Autodesk Fusion 360 part; units mm, degrees
note: some values were not read from the file. Set by a fixed rule: which sketch regions a step uses.
(part 3 of 3)
  point P196 (12, -62.3538)
  point P197 (12, -62.3538)
  point P198 (24, -62.3538)
  point P199 (24, -62.3538)
  point P200 (26.5, -58.0237)
  point P201 (29, -62.3538)
  point P202 (24, -62.3538)
  point P203 (24, -62.3538)
  point P204 (36, -62.3538)
  point P205 (36, -62.3538)
  point P206 (38.5, -58.0237)
  point P207 (41, -62.3538)
  point P208 (36, -62.3538)
  point P209 (36, -62.3538)
  point P210 (48, -62.3538)
  point P211 (48, -62.3538)
  point P212 (50.5, -58.0237)
  point P213 (53, -62.3538)
  point P214 (48, -62.3538)
  point P215 (48, -62.3538)
  point P216 (60, -62.3538)
  point P217 (60, -62.3538)
  point P218 (62.5, -58.0237)
  point P219 (65, -62.3538)
  point P220 (60, -62.3538)
  point P221 (60, -62.3538)
  point P222 (72, -62.3538)
  point P223 (72, -62.3538)
  point P224 (74.5, -58.0237)
  point P225 (77, -62.3538)
  point P226 (72, -62.3538)
  point P227 (72, -62.3538)
  point P228 (-138, -51.9615)
  point P229 (-138, -51.9615)
  point P230 (-135.5, -47.6314)
  point P231 (-133, -51.9615)
  point P232 (-138, -51.9615)
  point P233 (-138, -51.9615)
  point P234 (-126, -51.9615)
  point P235 (-126, -51.9615)
  point P236 (-123.5, -47.6314)
  point P237 (-121, -51.9615)
  point P238 (-126, -51.9615)
  point P239 (-126, -51.9615)
  point P240 (-114, -51.9615)
  point P241 (-114, -51.9615)
  point P242 (-111.5, -47.6314)
  point P243 (-109, -51.9615)
  point P244 (-114, -51.9615)
  point P245 (-114, -51.9615)
  point P246 (-102, -51.9615)
  point P247 (-102, -51.9615)
  point P248 (-99.5, -47.6314)
  point P249 (-97, -51.9615)
  point P250 (-102, -51.9615)
  point P251 (-102, -51.9615)
  point P252 (-90, -51.9615)
  point P253 (-90, -51.9615)
  point P254 (-87.5, -47.6314)
  point P255 (-85, -51.9615)
  point P256 (-90, -51.9615)
  point P257 (-90, -51.9615)
  point P258 (-78, -51.9615)
  point P259 (-78, -51.9615)
  point P260 (-75.5, -47.6314)
  point P261 (-73, -51.9615)
  point P262 (-78, -51.9615)
  point P263 (-78, -51.9615)
  point P264 (-66, -51.9615)
  point P265 (-66, -51.9615)
  point P266 (-63.5, -47.6314)
  point P267 (-61, -51.9615)
  point P268 (-66, -51.9615)
  point P269 (-66, -51.9615)
  point P270 (-54, -51.9615)
  point P271 (-54, -51.9615)
  point P272 (-51.5, -47.6314)
  point P273 (-49, -51.9615)
  point P274 (-54, -51.9615)
  point P275 (-54, -51.9615)
  point P276 (-42, -51.9615)
  point P277 (-42, -51.9615)
  point P278 (-39.5, -47.6314)
  point P279 (-37, -51.9615)
  point P280 (-42, -51.9615)
  point P281 (-42, -51.9615)
  point P282 (-30, -51.9615)
  point P283 (-30, -51.9615)
  point P284 (-27.5, -47.6314)
  point P285 (-25, -51.9615)
  point P286 (-30, -51.9615)
  point P287 (-30, -51.9615)
  point P288 (-18, -51.9615)
  point P289 (-18, -51.9615)
  point P290 (-15.5, -47.6314)
  point P291 (-13, -51.9615)
  point P292 (-18, -51.9615)
  point P293 (-18, -51.9615)
  point P294 (-6, -51.9615)
  point P295 (-6, -51.9615)
  point P296 (-3.5, -47.6314)
  point P297 (-1, -51.9615)
  point P298 (-6, -51.9615)
  point P299 (-6, -51.9615)
  point P300 (6, -51.9615)
  point P301 (6, -51.9615)
  point P302 (8.5, -47.6314)
  point P303 (11, -51.9615)
  point P304 (6, -51.9615)
  point P305 (6, -51.9615)
  point P306 (18, -51.9615)
  point P307 (18, -51.9615)
  point P308 (20.5, -47.6314)
  point P309 (23, -51.9615)
  point P310 (18, -51.9615)
  point P311 (18, -51.9615)
  point P312 (30, -51.9615)
  point P313 (30, -51.9615)
  point P314 (32.5, -47.6314)
  point P315 (35, -51.9615)
  point P316 (30, -51.9615)
  point P317 (30, -51.9615)
  point P318 (42, -51.9615)
  point P319 (42, -51.9615)
  point P320 (44.5, -47.6314)
  point P321 (47, -51.9615)
  point P322 (42, -51.9615)
  point P323 (42, -51.9615)
  point P324 (54, -51.9615)
  point P325 (54, -51.9615)
  point P326 (56.5, -47.6314)
  point P327 (59, -51.9615)
  point P328 (54, -51.9615)
  point P329 (54, -51.9615)
  point P330 (66, -51.9615)
  point P331 (66, -51.9615)
  point P332 (68.5, -47.6314)
  point P333 (71, -51.9615)
  point P334 (66, -51.9615)
  point P335 (66, -51.9615)
  point P336 (78, -51.9615)
  point P337 (78, -51.9615)
  point P338 (80.5, -47.6314)
  point P339 (83, -51.9615)
  point P340 (78, -51.9615)
  point P341 (78, -51.9615)
  point P342 (-132, -41.5692)
  point P343 (-132, -41.5692)
  point P344 (-129.5, -37.2391)
  point P345 (-127, -41.5692)
  point P346 (-132, -41.5692)
  point P347 (-132, -41.5692)
  point P348 (-120, -41.5692)
  point P349 (-120, -41.5692)
  point P350 (-117.5, -37.2391)
  point P351 (-115, -41.5692)
  point P352 (-120, -41.5692)
  point P353 (-120, -41.5692)
  point P354 (-108, -41.5692)
  point P355 (-108, -41.5692)
  point P356 (-105.5, -37.2391)
  point P357 (-103, -41.5692)
  point P358 (-108, -41.5692)
  point P359 (-108, -41.5692)
  point P360 (-96, -41.5692)
  point P361 (-96, -41.5692)
  point P362 (-93.5, -37.2391)
  point P363 (-91, -41.5692)
  point P364 (-96, -41.5692)
  point P365 (-96, -41.5692)
  point P366 (-84, -41.5692)
  point P367 (-84, -41.5692)
  point P368 (-81.5, -37.2391)
  point P369 (-79, -41.5692)
  point P370 (-84, -41.5692)
  point P371 (-84, -41.5692)
  point P372 (-72, -41.5692)
  point P373 (-72, -41.5692)
  point P374 (-69.5, -37.2391)
  point P375 (-67, -41.5692)
  point P376 (-72, -41.5692)
  point P377 (-72, -41.5692)
  point P378 (-60, -41.5692)
  point P379 (-60, -41.5692)
  point P380 (-57.5, -37.2391)
  point P381 (-55, -41.5692)
  point P382 (-60, -41.5692)
  point P383 (-60, -41.5692)
  point P384 (-48, -41.5692)
  point P385 (-48, -41.5692)
  point P386 (-45.5, -37.2391)
  point P387 (-43, -41.5692)
  point P388 (-48, -41.5692)
  point P389 (-48, -41.5692)
  point P390 (-36, -41.5692)
  point P391 (-36, -41.5692)
  point P392 (-33.5, -37.2391)
  point P393 (-31, -41.5692)
  point P394 (-36, -41.5692)
  point P395 (-36, -41.5692)
  point P396 (-24, -41.5692)
  point P397 (-24, -41.5692)
  point P398 (-21.5, -37.2391)
  point P399 (-19, -41.5692)
  point P400 (-24, -41.5692)
  point P401 (-24, -41.5692)
  point P402 (-12, -41.5692)
  point P403 (-12, -41.5692)
  point P404 (-9.5, -37.2391)
  point P405 (-7, -41.5692)
  point P406 (-12, -41.5692)
  point P407 (-12, -41.5692)
  point P408 (0, -41.5692)
  point P409 (0, -41.5692)
  point P410 (2.5, -37.2391)
  point P411 (5, -41.5692)
  point P412 (0, -41.5692)
  point P413 (0, -41.5692)
  point P414 (12, -41.5692)
  point P415 (12, -41.5692)
  point P416 (14.5, -37.2391)
  point P417 (17, -41.5692)
  point P418 (12, -41.5692)
  point P419 (12, -41.5692)
  point P420 (24, -41.5692)
  point P421 (24, -41.5692)
  point P422 (26.5, -37.2391)
  point P423 (29, -41.5692)
  point P424 (24, -41.5692)
  point P425 (24, -41.5692)
  point P426 (36, -41.5692)
  point P427 (36, -41.5692)
  point P428 (38.5, -37.2391)
  point P429 (41, -41.5692)
  point P430 (36, -41.5692)
  point P431 (36, -41.5692)
  point P432 (48, -41.5692)
  point P433 (48, -41.5692)
  point P434 (50.5, -37.2391)
  point P435 (53, -41.5692)
  point P436 (48, -41.5692)
  point P437 (48, -41.5692)
  point P438 (60, -41.5692)
  point P439 (60, -41.5692)
  point P440 (62.5, -37.2391)
  point P441 (65, -41.5692)
  point P442 (60, -41.5692)
  point P443 (60, -41.5692)
  point P444 (72, -41.5692)
  point P445 (72, -41.5692)
  point P446 (74.5, -37.2391)
  point P447 (77, -41.5692)
  point P448 (72, -41.5692)
  point P449 (72, -41.5692)
  point P450 (84, -41.5692)
  point P451 (84, -41.5692)
  point P452 (86.5, -37.2391)
  point P453 (89, -41.5692)
  point P454 (84, -41.5692)
  point P455 (84, -41.5692)
  point P456 (-126, -31.1769)
  point P457 (-126, -31.1769)
  point P458 (-123.5, -26.8468)
  point P459 (-121, -31.1769)
  point P460 (-126, -31.1769)
  point P461 (-126, -31.1769)
  point P462 (-114, -31.1769)
  point P463 (-114, -31.1769)
  point P464 (-111.5, -26.8468)
  point P465 (-109, -31.1769)
  point P466 (-114, -31.1769)
  point P467 (-114, -31.1769)
  point P468 (-102, -31.1769)
  point P469 (-102, -31.1769)
  point P470 (-99.5, -26.8468)
  point P471 (-97, -31.1769)
  point P472 (-102, -31.1769)
  point P473 (-102, -31.1769)
  point P474 (-90, -31.1769)
  point P475 (-90, -31.1769)
  point P476 (-87.5, -26.8468)
  point P477 (-85, -31.1769)
  point P478 (-90, -31.1769)
  point P479 (-90, -31.1769)
  point P480 (-78, -31.1769)
  point P481 (-78, -31.1769)
  point P482 (-75.5, -26.8468)
  point P483 (-73, -31.1769)
  point P484 (-78, -31.1769)
  point P485 (-78, -31.1769)
  point P486 (-66, -31.1769)
  point P487 (-66, -31.1769)
  point P488 (-63.5, -26.8468)
  point P489 (-61, -31.1769)
  point P490 (-66, -31.1769)
  point P491 (-66, -31.1769)
  point P492 (-54, -31.1769)
  point P493 (-54, -31.1769)
  point P494 (-51.5, -26.8468)
  point P495 (-49, -31.1769)
  point P496 (-54, -31.1769)
  point P497 (-54, -31.1769)
  point P498 (-42, -31.1769)
  point P499 (-42, -31.1769)
  point P500 (-39.5, -26.8468)
  point P501 (-37, -31.1769)
  point P502 (-42, -31.1769)
  point P503 (-42, -31.1769)
  point P504 (-30, -31.1769)
  point P505 (-30, -31.1769)
  point P506 (-27.5, -26.8468)
  point P507 (-25, -31.1769)
  point P508 (-30, -31.1769)
  point P509 (-30, -31.1769)
  point P510 (-18, -31.1769)
  point P511 (-18, -31.1769)
  point P512 (-15.5, -26.8468)
  point P513 (-13, -31.1769)
  point P514 (-18, -31.1769)
  point P515 (-18, -31.1769)
  point P516 (-6, -31.1769)
  point P517 (-6, -31.1769)
  point P518 (-3.5, -26.8468)
  point P519 (-1, -31.1769)
  point P520 (-6, -31.1769)
  point P521 (-6, -31.1769)
  point P522 (6, -31.1769)
  point P523 (6, -31.1769)
  point P524 (8.5, -26.8468)
  point P525 (11, -31.1769)
  point P526 (6, -31.1769)
  point P527 (6, -31.1769)
  point P528 (18, -31.1769)
  point P529 (18, -31.1769)
  point P530 (20.5, -26.8468)
  point P531 (23, -31.1769)
  point P532 (18, -31.1769)
  point P533 (18, -31.1769)
  point P534 (30, -31.1769)
  point P535 (30, -31.1769)
  point P536 (32.5, -26.8468)
  point P537 (35, -31.1769)
  point P538 (30, -31.1769)
  point P539 (30, -31.1769)
  point P540 (42, -31.1769)
  point P541 (42, -31.1769)
  point P542 (44.5, -26.8468)
  point P543 (47, -31.1769)
  point P544 (42, -31.1769)
  point P545 (42, -31.1769)
  point P546 (54, -31.1769)
  point P547 (54, -31.1769)
  point P548 (56.5, -26.8468)
  point P549 (59, -31.1769)
  point P550 (54, -31.1769)
  point P551 (54, -31.1769)
  point P552 (66, -31.1769)
  point P553 (66, -31.1769)
  point P554 (68.5, -26.8468)
  point P555 (71, -31.1769)
  point P556 (66, -31.1769)
  point P557 (66, -31.1769)
  point P558 (78, -31.1769)
  point P559 (78, -31.1769)
  point P560 (80.5, -26.8468)
  point P561 (83, -31.1769)
  point P562 (78, -31.1769)
  point P563 (78, -31.1769)
  point P564 (90, -31.1769)
  point P565 (90, -31.1769)
  point P566 (92.5, -26.8468)
  point P567 (95, -31.1769)
  point P568 (90, -31.1769)
  point P569 (90, -31.1769)
  point P570 (-120, -20.7846)
  point P571 (-120, -20.7846)
  point P572 (-117.5, -16.4545)
  point P573 (-115, -20.7846)
  point P574 (-120, -20.7846)
  point P575 (-120, -20.7846)
  point P576 (-108, -20.7846)
  point P577 (-108, -20.7846)
  point P578 (-105.5, -16.4545)
  point P579 (-103, -20.7846)
  point P580 (-108, -20.7846)
  point P581 (-108, -20.7846)
  point P582 (-96, -20.7846)
  point P583 (-96, -20.7846)
  point P584 (-93.5, -16.4545)
  point P585 (-91, -20.7846)
  point P586 (-96, -20.7846)
  point P587 (-96, -20.7846)
  point P588 (-84, -20.7846)
  point P589 (-84, -20.7846)
  point P590 (-81.5, -16.4545)
  point P591 (-79, -20.7846)
  point P592 (-84, -20.7846)
  point P593 (-84, -20.7846)
  point P594 (-72, -20.7846)
  point P595 (-72, -20.7846)
  point P596 (-69.5, -16.4545)
  point P597 (-67, -20.7846)
  point P598 (-72, -20.7846)
  point P599 (-72, -20.7846)
  point P600 (-60, -20.7846)
  point P601 (-60, -20.7846)
  point P602 (-57.5, -16.4545)
  point P603 (-55, -20.7846)
  point P604 (-60, -20.7846)
  point P605 (-60, -20.7846)
  point P606 (-48, -20.7846)
  point P607 (-48, -20.7846)
  point P608 (-45.5, -16.4545)
  point P609 (-43, -20.7846)
  point P610 (-48, -20.7846)
  point P611 (-48, -20.7846)
  point P612 (-36, -20.7846)
  point P613 (-36, -20.7846)
  point P614 (-33.5, -16.4545)
  point P615 (-31, -20.7846)
  point P616 (-36, -20.7846)
  point P617 (-36, -20.7846)
  point P618 (-24, -20.7846)
  point P619 (-24, -20.7846)
  point P620 (-21.5, -16.4545)
  point P621 (-19, -20.7846)
  point P622 (-24, -20.7846)
  point P623 (-24, -20.7846)
  point P624 (-12, -20.7846)
  point P625 (-12, -20.7846)
  point P626 (-9.5, -16.4545)
  point P627 (-7, -20.7846)
  point P628 (-12, -20.7846)
  point P629 (-12, -20.7846)
  point P630 (0, -20.7846)
  point P631 (0, -20.7846)
  point P632 (2.5, -16.4545)
  point P633 (5, -20.7846)
  point P634 (0, -20.7846)
  point P635 (0, -20.7846)
  point P636 (12, -20.7846)
  point P637 (12, -20.7846)
  point P638 (14.5, -16.4545)
  point P639 (17, -20.7846)
  point P640 (12, -20.7846)
  point P641 (12, -20.7846)
  point P642 (24, -20.7846)
  point P643 (24, -20.7846)
  point P644 (26.5, -16.4545)
  point P645 (29, -20.7846)
  point P646 (24, -20.7846)
  point P647 (24, -20.7846)
  point P648 (36, -20.7846)
  point P649 (36, -20.7846)
  point P650 (38.5, -16.4545)
  point P651 (41, -20.7846)
  point P652 (36, -20.7846)
  point P653 (36, -20.7846)
  point P654 (48, -20.7846)
  point P655 (48, -20.7846)
  point P656 (50.5, -16.4545)
  point P657 (53, -20.7846)
  point P658 (48, -20.7846)
  point P659 (48, -20.7846)
  point P660 (60, -20.7846)
  point P661 (60, -20.7846)
  point P662 (62.5, -16.4545)
  point P663 (65, -20.7846)
  point P664 (60, -20.7846)
  point P665 (60, -20.7846)
  point P666 (72, -20.7846)
  point P667 (72, -20.7846)
  point P668 (74.5, -16.4545)
  point P669 (77, -20.7846)
  point P670 (72, -20.7846)
  point P671 (72, -20.7846)
  point P672 (84, -20.7846)
  point P673 (84, -20.7846)
  point P674 (86.5, -16.4545)
  point P675 (89, -20.7846)
  point P676 (84, -20.7846)
  point P677 (84, -20.7846)
  point P678 (96, -20.7846)
  point P679 (96, -20.7846)
  point P680 (98.5, -16.4545)
  point P681 (101, -20.7846)
  point P682 (96, -20.7846)
  point P683 (96, -20.7846)
  point P684 (-114, -10.3923)
  point P685 (-114, -10.3923)
  point P686 (-111.5, -6.0622)
  point P687 (-109, -10.3923)
  point P688 (-114, -10.3923)
  point P689 (-114, -10.3923)
  point P690 (-102, -10.3923)
  point P691 (-102, -10.3923)
  point P692 (-99.5, -6.0622)
  point P693 (-97, -10.3923)
  point P694 (-102, -10.3923)
  point P695 (-102, -10.3923)
  point P696 (-90, -10.3923)
  point P697 (-90, -10.3923)
  point P698 (-87.5, -6.0622)
  point P699 (-85, -10.3923)
  point P700 (-90, -10.3923)
  point P701 (-90, -10.3923)
  point P702 (-78, -10.3923)
  point P703 (-78, -10.3923)
  point P704 (-75.5, -6.0622)
  point P705 (-73, -10.3923)
  point P706 (-78, -10.3923)
  point P707 (-78, -10.3923)
  point P708 (-66, -10.3923)
  point P709 (-66, -10.3923)
  point P710 (-63.5, -6.0622)
  point P711 (-61, -10.3923)
  point P712 (-66, -10.3923)
  point P713 (-66, -10.3923)
  point P714 (-54, -10.3923)
  point P715 (-54, -10.3923)
  point P716 (-51.5, -6.0622)
  point P717 (-49, -10.3923)
  point P718 (-54, -10.3923)
  point P719 (-54, -10.3923)
  point P720 (-42, -10.3923)
  point P721 (-42, -10.3923)
  point P722 (-39.5, -6.0622)
  point P723 (-37, -10.3923)
  point P724 (-42, -10.3923)
  point P725 (-42, -10.3923)
  point P726 (-30, -10.3923)
  point P727 (-30, -10.3923)
  point P728 (-27.5, -6.0622)
  point P729 (-25, -10.3923)
  point P730 (-30, -10.3923)
  point P731 (-30, -10.3923)
  point P732 (-18, -10.3923)
  point P733 (-18, -10.3923)
  point P734 (-15.5, -6.0622)
  point P735 (-13, -10.3923)
  point P736 (-18, -10.3923)
  point P737 (-18, -10.3923)
  point P738 (-6, -10.3923)
  point P739 (-6, -10.3923)
  point P740 (-3.5, -6.0622)
  point P741 (-1, -10.3923)
  point P742 (-6, -10.3923)
  point P743 (-6, -10.3923)
  point P744 (6, -10.3923)
  point P745 (6, -10.3923)
  point P746 (8.5, -6.0622)
  point P747 (11, -10.3923)
  point P748 (6, -10.3923)
  point P749 (6, -10.3923)
  point P750 (18, -10.3923)
  point P751 (18, -10.3923)
  point P752 (20.5, -6.0622)
  point P753 (23, -10.3923)
  point P754 (18, -10.3923)
  point P755 (18, -10.3923)
  point P756 (30, -10.3923)
  point P757 (30, -10.3923)
  point P758 (32.5, -6.0622)
  point P759 (35, -10.3923)
  point P760 (30, -10.3923)
  point P761 (30, -10.3923)
  point P762 (42, -10.3923)
  point P763 (42, -10.3923)
  point P764 (44.5, -6.0622)
  point P765 (47, -10.3923)
  point P766 (42, -10.3923)
  point P767 (42, -10.3923)
  point P768 (54, -10.3923)
  point P769 (54, -10.3923)
  point P770 (56.5, -6.0622)
  point P771 (59, -10.3923)
  point P772 (54, -10.3923)
  point P773 (54, -10.3923)
  point P774 (66, -10.3923)
  point P775 (66, -10.3923)
  point P776 (68.5, -6.0622)
  point P777 (71, -10.3923)
  point P778 (66, -10.3923)
  point P779 (66, -10.3923)
  point P780 (78, -10.3923)
  point P781 (78, -10.3923)
  point P782 (80.5, -6.0622)
  point P783 (83, -10.3923)
  point P784 (78, -10.3923)
  point P785 (78, -10.3923)
  point P786 (90, -10.3923)
  point P787 (90, -10.3923)
  point P788 (92.5, -6.0622)
  point P789 (95, -10.3923)
  point P790 (90, -10.3923)
  point P791 (90, -10.3923)
  point P792 (102, -10.3923)
  point P793 (102, -10.3923)
  point P794 (104.5, -6.0622)
  point P795 (107, -10.3923)
  point P796 (102, -10.3923)
  point P797 (102, -10.3923)
  point P798 (-108, 0)
  point P799 (-108, 0)
  point P800 (-105.5, 4.3301)
  point P801 (-103, 0)
  point P802 (-108, 0)
  point P803 (-108, 0)
  point P804 (-96, 0)
  point P805 (-96, 0)
  point P806 (-93.5, 4.3301)
  point P807 (-91, 0)
  point P808 (-96, 0)
  point P809 (-96, 0)
  point P810 (-84, 0)
  point P811 (-84, 0)
  point P812 (-81.5, 4.3301)
  point P813 (-79, 0)
  point P814 (-84, 0)
  point P815 (-84, 0)
  point P816 (-72, 0)
  point P817 (-72, 0)
  point P818 (-69.5, 4.3301)
  point P819 (-67, 0)
  point P820 (-72, 0)
  point P821 (-72, 0)
  point P822 (-60, 0)
  point P823 (-60, 0)
  point P824 (-57.5, 4.3301)
  point P825 (-55, 0)
  point P826 (-60, 0)
  point P827 (-60, 0)
  point P828 (-48, 0)
  point P829 (-48, 0)
  point P830 (-45.5, 4.3301)
  point P831 (-43, 0)
  point P832 (-48, 0)
  point P833 (-48, 0)
  point P834 (-36, 0)
  point P835 (-36, 0)
  point P836 (-33.5, 4.3301)
  point P837 (-31, 0)
  point P838 (-36, 0)
  point P839 (-36, 0)
  point P840 (-24, 0)
  point P841 (-24, 0)
  point P842 (-21.5, 4.3301)
  point P843 (-19, 0)
  point P844 (-24, 0)
  point P845 (-24, 0)
  point P846 (-12, 0)
  point P847 (-12, 0)
  point P848 (-9.5, 4.3301)
  point P849 (-7, 0)
  point P850 (-12, 0)
  point P851 (-12, 0)
  point P852 (12, 0)
  point P853 (12, 0)
  point P854 (14.5, 4.3301)
  point P855 (17, 0)
  point P856 (12, 0)
  point P857 (12, 0)
  point P858 (24, 0)
  point P859 (24, 0)
  point P860 (26.5, 4.3301)
  point P861 (29, 0)
  point P862 (24, 0)
  point P863 (24, 0)
  point P864 (36, 0)
  point P865 (36, 0)
  point P866 (38.5, 4.3301)
  point P867 (41, 0)
  point P868 (36, 0)
  point P869 (36, 0)
  point P870 (48, 0)
  point P871 (48, 0)
  point P872 (50.5, 4.3301)
  point P873 (53, 0)
  point P874 (48, 0)
  point P875 (48, 0)
  point P876 (60, 0)
  point P877 (60, 0)
  point P878 (62.5, 4.3301)
  point P879 (65, 0)
  point P880 (60, 0)
  point P881 (60, 0)
  point P882 (72, 0)
  point P883 (72, 0)
  point P884 (74.5, 4.3301)
  point P885 (77, 0)
  point P886 (72, 0)
  point P887 (72, 0)
  point P888 (84, 0)
  point P889 (84, 0)
  point P890 (86.5, 4.3301)
  point P891 (89, 0)
  point P892 (84, 0)
  point P893 (84, 0)
  point P894 (96, 0)
  point P895 (96, 0)
  point P896 (98.5, 4.3301)
  point P897 (101, 0)
  point P898 (96, 0)
  point P899 (96, 0)
  point P900 (108, 0)
  point P901 (108, 0)
  point P902 (110.5, 4.3301)
  point P903 (113, 0)
  point P904 (108, 0)
  point P905 (108, 0)
  point P906 (-102, 10.3923)
  point P907 (-102, 10.3923)
  point P908 (-99.5, 14.7224)
  point P909 (-97, 10.3923)
  point P910 (-102, 10.3923)
  point P911 (-102, 10.3923)
  point P912 (-90, 10.3923)
  point P913 (-90, 10.3923)
  point P914 (-87.5, 14.7224)
  point P915 (-85, 10.3923)
  point P916 (-90, 10.3923)
  point P917 (-90, 10.3923)
  point P918 (-78, 10.3923)
  point P919 (-78, 10.3923)
  point P920 (-75.5, 14.7224)
  point P921 (-73, 10.3923)
  point P922 (-78, 10.3923)
  point P923 (-78, 10.3923)
  point P924 (-66, 10.3923)
  point P925 (-66, 10.3923)
  point P926 (-63.5, 14.7224)
  point P927 (-61, 10.3923)
  point P928 (-66, 10.3923)
  point P929 (-66, 10.3923)
  point P930 (-54, 10.3923)
  point P931 (-54, 10.3923)
  point P932 (-51.5, 14.7224)
  point P933 (-49, 10.3923)
  point P934 (-54, 10.3923)
  point P935 (-54, 10.3923)
  point P936 (-42, 10.3923)
  point P937 (-42, 10.3923)
  point P938 (-39.5, 14.7224)
  point P939 (-37, 10.3923)
  point P940 (-42, 10.3923)
  point P941 (-42, 10.3923)
  point P942 (-30, 10.3923)
  point P943 (-30, 10.3923)
  point P944 (-27.5, 14.7224)
  point P945 (-25, 10.3923)
  point P946 (-30, 10.3923)
  point P947 (-30, 10.3923)
  point P948 (-18, 10.3923)
  point P949 (-18, 10.3923)
  point P950 (-15.5, 14.7224)
  point P951 (-13, 10.3923)
  point P952 (-18, 10.3923)
  point P953 (-18, 10.3923)
  point P954 (-6, 10.3923)
  point P955 (-6, 10.3923)
  point P956 (-3.5, 14.7224)
  point P957 (-1, 10.3923)
  point P958 (-6, 10.3923)
  point P959 (-6, 10.3923)
  point P960 (6, 10.3923)
  point P961 (6, 10.3923)
  point P962 (8.5, 14.7224)
  point P963 (11, 10.3923)
  point P964 (6, 10.3923)
  point P965 (6, 10.3923)
  point P966 (18, 10.3923)
  point P967 (18, 10.3923)
  point P968 (20.5, 14.7224)
  point P969 (23, 10.3923)
  point P970 (18, 10.3923)
  point P971 (18, 10.3923)
  point P972 (30, 10.3923)
  point P973 (30, 10.3923)
  point P974 (32.5, 14.7224)
  point P975 (35, 10.3923)
  point P976 (30, 10.3923)
  point P977 (30, 10.3923)
  point P978 (42, 10.3923)
  point P979 (42, 10.3923)
  point P980 (44.5, 14.7224)
  point P981 (47, 10.3923)
  point P982 (42, 10.3923)
  point P983 (42, 10.3923)
  point P984 (54, 10.3923)
  point P985 (54, 10.3923)
  point P986 (56.5, 14.7224)
  point P987 (59, 10.3923)
  point P988 (54, 10.3923)
  point P989 (54, 10.3923)
  point P990 (66, 10.3923)
  point P991 (66, 10.3923)
  point P992 (68.5, 14.7224)
  point P993 (71, 10.3923)
  point P994 (66, 10.3923)
  point P995 (66, 10.3923)
  point P996 (78, 10.3923)
  point P997 (78, 10.3923)
  point P998 (80.5, 14.7224)
  point P999 (83, 10.3923)
  point P1000 (78, 10.3923)
  point P1001 (78, 10.3923)
  point P1002 (90, 10.3923)
  point P1003 (90, 10.3923)
  point P1004 (92.5, 14.7224)
  point P1005 (95, 10.3923)
  point P1006 (90, 10.3923)
  point P1007 (90, 10.3923)
  point P1008 (102, 10.3923)
  point P1009 (102, 10.3923)
  point P1010 (104.5, 14.7224)
  point P1011 (107, 10.3923)
  point P1012 (102, 10.3923)
  point P1013 (102, 10.3923)
  point P1014 (114, 10.3923)
  point P1015 (114, 10.3923)
  point P1016 (116.5, 14.7224)
  point P1017 (119, 10.3923)
  point P1018 (114, 10.3923)
  point P1019 (114, 10.3923)
  point P1020 (-96, 20.7846)
  point P1021 (-96, 20.7846)
  point P1022 (-93.5, 25.1147)
  point P1023 (-91, 20.7846)
  point P1024 (-96, 20.7846)
  point P1025 (-96, 20.7846)
  point P1026 (-84, 20.7846)
  point P1027 (-84, 20.7846)
  point P1028 (-81.5, 25.1147)
  point P1029 (-79, 20.7846)
  point P1030 (-84, 20.7846)
  point P1031 (-84, 20.7846)
  point P1032 (-72, 20.7846)
  point P1033 (-72, 20.7846)
  point P1034 (-69.5, 25.1147)
  point P1035 (-67, 20.7846)
  point P1036 (-72, 20.7846)
  point P1037 (-72, 20.7846)
  point P1038 (-60, 20.7846)
  point P1039 (-60, 20.7846)
  point P1040 (-57.5, 25.1147)
  point P1041 (-55, 20.7846)
  point P1042 (-60, 20.7846)
  point P1043 (-60, 20.7846)
  point P1044 (-48, 20.7846)
  point P1045 (-48, 20.7846)
  point P1046 (-45.5, 25.1147)
  point P1047 (-43, 20.7846)
  point P1048 (-48, 20.7846)
  point P1049 (-48, 20.7846)
  point P1050 (-36, 20.7846)
  point P1051 (-36, 20.7846)
  point P1052 (-33.5, 25.1147)
  point P1053 (-31, 20.7846)
  point P1054 (-36, 20.7846)
  point P1055 (-36, 20.7846)
  point P1056 (-24, 20.7846)
  point P1057 (-24, 20.7846)
  point P1058 (-21.5, 25.1147)
  point P1059 (-19, 20.7846)
  point P1060 (-24, 20.7846)
  point P1061 (-24, 20.7846)
  point P1062 (-12, 20.7846)
  point P1063 (-12, 20.7846)
  point P1064 (-9.5, 25.1147)
  point P1065 (-7, 20.7846)
  point P1066 (-12, 20.7846)
  point P1067 (-12, 20.7846)
  point P1068 (0, 20.7846)
  point P1069 (0, 20.7846)
  point P1070 (2.5, 25.1147)
  point P1071 (5, 20.7846)
  point P1072 (0, 20.7846)
  point P1073 (0, 20.7846)
  point P1074 (12, 20.7846)
  point P1075 (12, 20.7846)
  point P1076 (14.5, 25.1147)
  point P1077 (17, 20.7846)
  point P1078 (12, 20.7846)
  point P1079 (12, 20.7846)
  point P1080 (24, 20.7846)
  point P1081 (24, 20.7846)
  point P1082 (26.5, 25.1147)
  point P1083 (29, 20.7846)
  point P1084 (24, 20.7846)
  point P1085 (24, 20.7846)
  point P1086 (36, 20.7846)
  point P1087 (36, 20.7846)
  point P1088 (38.5, 25.1147)
  point P1089 (41, 20.7846)
  point P1090 (36, 20.7846)
  point P1091 (36, 20.7846)
  point P1092 (48, 20.7846)
  point P1093 (48, 20.7846)
  point P1094 (50.5, 25.1147)
  point P1095 (53, 20.7846)
  point P1096 (48, 20.7846)
  point P1097 (48, 20.7846)
  point P1098 (60, 20.7846)
  point P1099 (60, 20.7846)
  point P1100 (62.5, 25.1147)
  point P1101 (65, 20.7846)
  point P1102 (60, 20.7846)
  point P1103 (60, 20.7846)
  point P1104 (72, 20.7846)
  point P1105 (72, 20.7846)
  point P1106 (74.5, 25.1147)
  point P1107 (77, 20.7846)
  point P1108 (72, 20.7846)
  point P1109 (72, 20.7846)
  point P1110 (84, 20.7846)
  point P1111 (84, 20.7846)
  point P1112 (86.5, 25.1147)
  point P1113 (89, 20.7846)
  point P1114 (84, 20.7846)
  point P1115 (84, 20.7846)
  point P1116 (96, 20.7846)
  point P1117 (96, 20.7846)
  point P1118 (98.5, 25.1147)
  point P1119 (101, 20.7846)
  point P1120 (96, 20.7846)
  point P1121 (96, 20.7846)
  point P1122 (108, 20.7846)
  point P1123 (108, 20.7846)
  point P1124 (110.5, 25.1147)
  point P1125 (113, 20.7846)
  point P1126 (108, 20.7846)
  point P1127 (108, 20.7846)
  point P1128 (120, 20.7846)
  point P1129 (120, 20.7846)
  point P1130 (122.5, 25.1147)
  point P1131 (125, 20.7846)
  point P1132 (120, 20.7846)
  point P1133 (120, 20.7846)
  point P1134 (-90, 31.1769)
  point P1135 (-90, 31.1769)
  point P1136 (-87.5, 35.507)
  point P1137 (-85, 31.1769)
  point P1138 (-90, 31.1769)
  point P1139 (-90, 31.1769)
  point P1140 (-78, 31.1769)
  point P1141 (-78, 31.1769)
  point P1142 (-75.5, 35.507)
  point P1143 (-73, 31.1769)
  point P1144 (-78, 31.1769)
  point P1145 (-78, 31.1769)
  point P1146 (-66, 31.1769)
  point P1147 (-66, 31.1769)
  point P1148 (-63.5, 35.507)
  point P1149 (-61, 31.1769)
  point P1150 (-66, 31.1769)
  point P1151 (-66, 31.1769)
  point P1152 (-54, 31.1769)
  point P1153 (-54, 31.1769)
  point P1154 (-51.5, 35.507)
  point P1155 (-49, 31.1769)
  point P1156 (-54, 31.1769)
  point P1157 (-54, 31.1769)
  point P1158 (-42, 31.1769)
  point P1159 (-42, 31.1769)
  point P1160 (-39.5, 35.507)
  point P1161 (-37, 31.1769)
  point P1162 (-42, 31.1769)
  point P1163 (-42, 31.1769)
  point P1164 (-30, 31.1769)
  point P1165 (-30, 31.1769)
  point P1166 (-27.5, 35.507)
  point P1167 (-25, 31.1769)
  point P1168 (-30, 31.1769)
  point P1169 (-30, 31.1769)
  point P1170 (-18, 31.1769)
  point P1171 (-18, 31.1769)
  point P1172 (-15.5, 35.507)
  point P1173 (-13, 31.1769)
  point P1174 (-18, 31.1769)
  point P1175 (-18, 31.1769)
  point P1176 (-6, 31.1769)
  point P1177 (-6, 31.1769)
  point P1178 (-3.5, 35.507)
  point P1179 (-1, 31.1769)
  point P1180 (-6, 31.1769)
  point P1181 (-6, 31.1769)
  point P1182 (6, 31.1769)
  point P1183 (6, 31.1769)
  point P1184 (8.5, 35.507)
  point P1185 (11, 31.1769)
  point P1186 (6, 31.1769)
  point P1187 (6, 31.1769)
  point P1188 (18, 31.1769)
  point P1189 (18, 31.1769)
  point P1190 (20.5, 35.507)
  point P1191 (23, 31.1769)
  point P1192 (18, 31.1769)
  point P1193 (18, 31.1769)
  point P1194 (30, 31.1769)
  point P1195 (30, 31.1769)
  point P1196 (32.5, 35.507)
  point P1197 (35, 31.1769)
  point P1198 (30, 31.1769)
  point P1199 (30, 31.1769)
  point P1200 (42, 31.1769)
  point P1201 (42, 31.1769)
  point P1202 (44.5, 35.507)
  point P1203 (47, 31.1769)
  point P1204 (42, 31.1769)
  point P1205 (42, 31.1769)
  point P1206 (54, 31.1769)
  point P1207 (54, 31.1769)
  point P1208 (56.5, 35.507)
  point P1209 (59, 31.1769)
  point P1210 (54, 31.1769)
  point P1211 (54, 31.1769)
  point P1212 (66, 31.1769)
  point P1213 (66, 31.1769)
  point P1214 (68.5, 35.507)
  point P1215 (71, 31.1769)
  point P1216 (66, 31.1769)
  point P1217 (66, 31.1769)
  point P1218 (78, 31.1769)
  point P1219 (78, 31.1769)
  point P1220 (80.5, 35.507)
  point P1221 (83, 31.1769)
  point P1222 (78, 31.1769)
  point P1223 (78, 31.1769)
  point P1224 (90, 31.1769)
  point P1225 (90, 31.1769)
  point P1226 (92.5, 35.507)
  point P1227 (95, 31.1769)
  point P1228 (90, 31.1769)
  point P1229 (90, 31.1769)
  point P1230 (102, 31.1769)
  point P1231 (102, 31.1769)
  point P1232 (104.5, 35.507)
  point P1233 (107, 31.1769)
  point P1234 (102, 31.1769)
  point P1235 (102, 31.1769)
  point P1236 (114, 31.1769)
  point P1237 (114, 31.1769)
  point P1238 (116.5, 35.507)
  point P1239 (119, 31.1769)
  point P1240 (114, 31.1769)
  point P1241 (114, 31.1769)
  point P1242 (126, 31.1769)
  point P1243 (126, 31.1769)
  point P1244 (128.5, 35.507)
  point P1245 (131, 31.1769)
  point P1246 (126, 31.1769)
  point P1247 (126, 31.1769)
  point P1248 (-84, 41.5692)
  point P1249 (-84, 41.5692)
  point P1250 (-81.5, 45.8993)
  point P1251 (-79, 41.5692)
  point P1252 (-84, 41.5692)
  point P1253 (-84, 41.5692)
  point P1254 (-72, 41.5692)
  point P1255 (-72, 41.5692)
  point P1256 (-69.5, 45.8993)
  point P1257 (-67, 41.5692)
  point P1258 (-72, 41.5692)
  point P1259 (-72, 41.5692)
  point P1260 (-60, 41.5692)
  point P1261 (-60, 41.5692)
  point P1262 (-57.5, 45.8993)
  point P1263 (-55, 41.5692)
  point P1264 (-60, 41.5692)
  point P1265 (-60, 41.5692)
  point P1266 (-48, 41.5692)
  point P1267 (-48, 41.5692)
  point P1268 (-45.5, 45.8993)
  point P1269 (-43, 41.5692)
  point P1270 (-48, 41.5692)
  point P1271 (-48, 41.5692)
  point P1272 (-36, 41.5692)
  point P1273 (-36, 41.5692)
  point P1274 (-33.5, 45.8993)
  point P1275 (-31, 41.5692)
  point P1276 (-36, 41.5692)
  point P1277 (-36, 41.5692)
  point P1278 (-24, 41.5692)
  point P1279 (-24, 41.5692)
  point P1280 (-21.5, 45.8993)
  point P1281 (-19, 41.5692)
  point P1282 (-24, 41.5692)
  point P1283 (-24, 41.5692)
  point P1284 (-12, 41.5692)
  point P1285 (-12, 41.5692)
  point P1286 (-9.5, 45.8993)
  point P1287 (-7, 41.5692)
  point P1288 (-12, 41.5692)
  point P1289 (-12, 41.5692)
  point P1290 (0, 41.5692)
  point P1291 (0, 41.5692)
  point P1292 (2.5, 45.8993)
  point P1293 (5, 41.5692)
  point P1294 (0, 41.5692)
  point P1295 (0, 41.5692)
  point P1296 (12, 41.5692)
  point P1297 (12, 41.5692)
  point P1298 (14.5, 45.8993)
  point P1299 (17, 41.5692)
  point P1300 (12, 41.5692)
  point P1301 (12, 41.5692)
  point P1302 (24, 41.5692)
  point P1303 (24, 41.5692)
  point P1304 (26.5, 45.8993)
  point P1305 (29, 41.5692)
  point P1306 (24, 41.5692)
  point P1307 (24, 41.5692)
  point P1308 (36, 41.5692)
  point P1309 (36, 41.5692)
  point P1310 (38.5, 45.8993)
  point P1311 (41, 41.5692)
  point P1312 (36, 41.5692)
  point P1313 (36, 41.5692)
  point P1314 (48, 41.5692)
  point P1315 (48, 41.5692)
  point P1316 (50.5, 45.8993)
  point P1317 (53, 41.5692)
  point P1318 (48, 41.5692)
  point P1319 (48, 41.5692)
  point P1320 (60, 41.5692)
  point P1321 (60, 41.5692)
  point P1322 (62.5, 45.8993)
  point P1323 (65, 41.5692)
  point P1324 (60, 41.5692)
  point P1325 (60, 41.5692)
  point P1326 (72, 41.5692)
  point P1327 (72, 41.5692)
  point P1328 (74.5, 45.8993)
  point P1329 (77, 41.5692)
  point P1330 (72, 41.5692)
  point P1331 (72, 41.5692)
  point P1332 (84, 41.5692)
  point P1333 (84, 41.5692)
  point P1334 (86.5, 45.8993)
  point P1335 (89, 41.5692)
  point P1336 (84, 41.5692)
  point P1337 (84, 41.5692)
  point P1338 (96, 41.5692)
  point P1339 (96, 41.5692)
  point P1340 (98.5, 45.8993)
  point P1341 (101, 41.5692)
  point P1342 (96, 41.5692)
  point P1343 (96, 41.5692)
  point P1344 (108, 41.5692)
  point P1345 (108, 41.5692)
  point P1346 (110.5, 45.8993)
  point P1347 (113, 41.5692)
  point P1348 (108, 41.5692)
  point P1349 (108, 41.5692)
  point P1350 (120, 41.5692)
  point P1351 (120, 41.5692)
  point P1352 (122.5, 45.8993)
  point P1353 (125, 41.5692)
  point P1354 (120, 41.5692)
  point P1355 (120, 41.5692)
  point P1356 (132, 41.5692)
  point P1357 (132, 41.5692)
  point P1358 (134.5, 45.8993)
  point P1359 (137, 41.5692)
  point P1360 (132, 41.5692)
  point P1361 (132, 41.5692)
  point P1362 (-78, 51.9615)
  point P1363 (-78, 51.9615)
  point P1364 (-75.5, 56.2917)
  point P1365 (-73, 51.9615)
  point P1366 (-78, 51.9615)
  point P1367 (-78, 51.9615)
  point P1368 (-66, 51.9615)
  point P1369 (-66, 51.9615)
  point P1370 (-63.5, 56.2917)
  point P1371 (-61, 51.9615)
  point P1372 (-66, 51.9615)
  point P1373 (-66, 51.9615)
  point P1374 (-54, 51.9615)
  point P1375 (-54, 51.9615)
  point P1376 (-51.5, 56.2917)
  point P1377 (-49, 51.9615)
  point P1378 (-54, 51.9615)
  point P1379 (-54, 51.9615)
  point P1380 (-42, 51.9615)
  point P1381 (-42, 51.9615)
  point P1382 (-39.5, 56.2917)
  point P1383 (-37, 51.9615)
  point P1384 (-42, 51.9615)
  point P1385 (-42, 51.9615)
  point P1386 (-30, 51.9615)
  point P1387 (-30, 51.9615)
  point P1388 (-27.5, 56.2917)
  point P1389 (-25, 51.9615)
  point P1390 (-30, 51.9615)
  point P1391 (-30, 51.9615)
  point P1392 (-18, 51.9615)
  point P1393 (-18, 51.9615)
  point P1394 (-15.5, 56.2917)
  point P1395 (-13, 51.9615)
  point P1396 (-18, 51.9615)
  point P1397 (-18, 51.9615)
  point P1398 (-6, 51.9615)
  point P1399 (-6, 51.9615)
  point P1400 (-3.5, 56.2917)
  point P1401 (-1, 51.9615)
  point P1402 (-6, 51.9615)
  point P1403 (-6, 51.9615)
  point P1404 (6, 51.9615)
  point P1405 (6, 51.9615)
  point P1406 (8.5, 56.2917)
  point P1407 (11, 51.9615)
  point P1408 (6, 51.9615)
  point P1409 (6, 51.9615)
  point P1410 (18, 51.9615)
  point P1411 (18, 51.9615)
  point P1412 (20.5, 56.2917)
  point P1413 (23, 51.9615)
  point P1414 (18, 51.9615)
  point P1415 (18, 51.9615)
  point P1416 (30, 51.9615)
  point P1417 (30, 51.9615)
  point P1418 (32.5, 56.2917)
  point P1419 (35, 51.9615)
  point P1420 (30, 51.9615)
  point P1421 (30, 51.9615)
  point P1422 (42, 51.9615)
  point P1423 (42, 51.9615)
  point P1424 (44.5, 56.2917)
  point P1425 (47, 51.9615)
  point P1426 (42, 51.9615)
  point P1427 (42, 51.9615)
  point P1428 (54, 51.9615)
  point P1429 (54, 51.9615)
  point P1430 (56.5, 56.2917)
  point P1431 (59, 51.9615)
  point P1432 (54, 51.9615)
  point P1433 (54, 51.9615)
  point P1434 (66, 51.9615)
  point P1435 (66, 51.9615)
  point P1436 (68.5, 56.2917)
  point P1437 (71, 51.9615)
  point P1438 (66, 51.9615)
  point P1439 (66, 51.9615)
  point P1440 (78, 51.9615)
  point P1441 (78, 51.9615)
  point P1442 (80.5, 56.2917)
  point P1443 (83, 51.9615)
  point P1444 (78, 51.9615)
  point P1445 (78, 51.9615)
  point P1446 (90, 51.9615)
  point P1447 (90, 51.9615)
  point P1448 (92.5, 56.2917)
  point P1449 (95, 51.9615)
  point P1450 (90, 51.9615)
  point P1451 (90, 51.9615)
  point P1452 (102, 51.9615)
  point P1453 (102, 51.9615)
  point P1454 (104.5, 56.2917)
  point P1455 (107, 51.9615)
  point P1456 (102, 51.9615)
  point P1457 (102, 51.9615)
  point P1458 (114, 51.9615)
  point P1459 (114, 51.9615)
  point P1460 (116.5, 56.2917)
  point P1461 (119, 51.9615)
  point P1462 (114, 51.9615)
  point P1463 (114, 51.9615)
  point P1464 (126, 51.9615)
  point P1465 (126, 51.9615)
  point P1466 (128.5, 56.2917)
  point P1467 (131, 51.9615)
  point P1468 (126, 51.9615)
  point P1469 (126, 51.9615)
  point P1470 (138, 51.9615)
  point P1471 (138, 51.9615)
  point P1472 (140.5, 56.2917)
  point P1473 (143, 51.9615)
  point P1474 (138, 51.9615)
  point P1475 (138, 51.9615)
  point P1476 (-72, 62.3538)
  point P1477 (-72, 62.3538)
  point P1478 (-69.5, 66.684)
  point P1479 (-67, 62.3538)
  point P1480 (-72, 62.3538)
  point P1481 (-72, 62.3538)
  point P1482 (-60, 62.3538)
  point P1483 (-60, 62.3538)
  point P1484 (-57.5, 66.684)
  point P1485 (-55, 62.3538)
  point P1486 (-60, 62.3538)
  point P1487 (-60, 62.3538)
  point P1488 (-48, 62.3538)
  point P1489 (-48, 62.3538)
  point P1490 (-45.5, 66.684)
  point P1491 (-43, 62.3538)
  point P1492 (-48, 62.3538)
  point P1493 (-48, 62.3538)
  point P1494 (-36, 62.3538)
  point P1495 (-36, 62.3538)
  point P1496 (-33.5, 66.684)
  point P1497 (-31, 62.3538)
  point P1498 (-36, 62.3538)
  point P1499 (-36, 62.3538)
  point P1500 (-24, 62.3538)
  point P1501 (-24, 62.3538)
  point P1502 (-21.5, 66.684)
  point P1503 (-19, 62.3538)
  point P1504 (-24, 62.3538)
  point P1505 (-24, 62.3538)
  point P1506 (-12, 62.3538)
  point P1507 (-12, 62.3538)
  point P1508 (-9.5, 66.684)
  point P1509 (-7, 62.3538)
  point P1510 (-12, 62.3538)
  point P1511 (-12, 62.3538)
  point P1512 (0, 62.3538)
  point P1513 (0, 62.3538)
  point P1514 (2.5, 66.684)
  point P1515 (5, 62.3538)
  point P1516 (0, 62.3538)
  point P1517 (0, 62.3538)
  point P1518 (12, 62.3538)
  point P1519 (12, 62.3538)
  point P1520 (14.5, 66.684)
  point P1521 (17, 62.3538)
  point P1522 (12, 62.3538)
  point P1523 (12, 62.3538)
  point P1524 (24, 62.3538)
  point P1525 (24, 62.3538)
  point P1526 (26.5, 66.684)
  point P1527 (29, 62.3538)
  point P1528 (24, 62.3538)
  point P1529 (24, 62.3538)
  point P1530 (36, 62.3538)
  point P1531 (36, 62.3538)
  point P1532 (38.5, 66.684)
  point P1533 (41, 62.3538)
  point P1534 (36, 62.3538)
  point P1535 (36, 62.3538)
  point P1536 (48, 62.3538)
  point P1537 (48, 62.3538)
  point P1538 (50.5, 66.684)
  point P1539 (53, 62.3538)
  point P1540 (48, 62.3538)
  point P1541 (48, 62.3538)
  point P1542 (60, 62.3538)
  point P1543 (60, 62.3538)
  point P1544 (62.5, 66.684)
  point P1545 (65, 62.3538)
  point P1546 (60, 62.3538)
  point P1547 (60, 62.3538)
  point P1548 (72, 62.3538)
  point P1549 (72, 62.3538)
  point P1550 (74.5, 66.684)
  point P1551 (77, 62.3538)
  point P1552 (72, 62.3538)
  point P1553 (72, 62.3538)
  point P1554 (84, 62.3538)
  point P1555 (84, 62.3538)
  point P1556 (86.5, 66.684)
  point P1557 (89, 62.3538)
  point P1558 (84, 62.3538)
  point P1559 (84, 62.3538)
  point P1560 (96, 62.3538)
  point P1561 (96, 62.3538)
  point P1562 (98.5, 66.684)
  point P1563 (101, 62.3538)
  point P1564 (96, 62.3538)
  point P1565 (96, 62.3538)
  point P1566 (108, 62.3538)
  point P1567 (108, 62.3538)
  point P1568 (110.5, 66.684)
  point P1569 (113, 62.3538)
  point P1570 (108, 62.3538)
  point P1571 (108, 62.3538)
  point P1572 (120, 62.3538)
  point P1573 (120, 62.3538)
  point P1574 (122.5, 66.684)
  point P1575 (125, 62.3538)
  point P1576 (120, 62.3538)
  point P1577 (120, 62.3538)
  point P1578 (132, 62.3538)
  point P1579 (132, 62.3538)
  point P1580 (134.5, 66.684)
  point P1581 (137, 62.3538)
  point P1582 (132, 62.3538)
  point P1583 (132, 62.3538)
  point P1584 (144, 62.3538)
  point P1585 (144, 62.3538)
  point P1586 (146.5, 66.684)
  point P1587 (149, 62.3538)
  point P1588 (144, 62.3538)
  point P1589 (144, 62.3538)
  point P1590 (-66, 72.7461)
  point P1591 (-66, 72.7461)
  point P1592 (-63.5, 77.0763)
  point P1593 (-61, 72.7461)
  point P1594 (-66, 72.7461)
  point P1595 (-66, 72.7461)
  point P1596 (-54, 72.7461)
  point P1597 (-54, 72.7461)
  point P1598 (-51.5, 77.0763)
  point P1599 (-49, 72.7461)
  point P1600 (-54, 72.7461)
  point P1601 (-54, 72.7461)
  point P1602 (-42, 72.7461)
  point P1603 (-42, 72.7461)
  point P1604 (-39.5, 77.0763)
  point P1605 (-37, 72.7461)
  point P1606 (-42, 72.7461)
  point P1607 (-42, 72.7461)
  point P1608 (-30, 72.7461)
  point P1609 (-30, 72.7461)
  point P1610 (-27.5, 77.0763)
  point P1611 (-25, 72.7461)
  point P1612 (-30, 72.7461)
  point P1613 (-30, 72.7461)
  point P1614 (-18, 72.7461)
  point P1615 (-18, 72.7461)
  point P1616 (-15.5, 77.0763)
  point P1617 (-13, 72.7461)
  point P1618 (-18, 72.7461)
  point P1619 (-18, 72.7461)
  point P1620 (-6, 72.7461)
  point P1621 (-6, 72.7461)
  point P1622 (-3.5, 77.0763)
  point P1623 (-1, 72.7461)
  point P1624 (-6, 72.7461)
  point P1625 (-6, 72.7461)
  point P1626 (6, 72.7461)
  point P1627 (6, 72.7461)
  point P1628 (8.5, 77.0763)
  point P1629 (11, 72.7461)
  point P1630 (6, 72.7461)
  point P1631 (6, 72.7461)
  point P1632 (18, 72.7461)
  point P1633 (18, 72.7461)
  point P1634 (20.5, 77.0763)
  point P1635 (23, 72.7461)
  point P1636 (18, 72.7461)
  point P1637 (18, 72.7461)
  point P1638 (30, 72.7461)
  point P1639 (30, 72.7461)
  point P1640 (32.5, 77.0763)
  point P1641 (35, 72.7461)
  point P1642 (30, 72.7461)
  point P1643 (30, 72.7461)
  point P1644 (42, 72.7461)
  point P1645 (42, 72.7461)
  point P1646 (44.5, 77.0763)
  point P1647 (47, 72.7461)
  point P1648 (42, 72.7461)
  point P1649 (42, 72.7461)
  point P1650 (54, 72.7461)
  point P1651 (54, 72.7461)
  point P1652 (56.5, 77.0763)
  point P1653 (59, 72.7461)
  point P1654 (54, 72.7461)
  point P1655 (54, 72.7461)
  point P1656 (66, 72.7461)
  point P1657 (66, 72.7461)
  point P1658 (68.5, 77.0763)
  point P1659 (71, 72.7461)
  point P1660 (66, 72.7461)
  point P1661 (66, 72.7461)
  point P1662 (78, 72.7461)
  point P1663 (78, 72.7461)
  point P1664 (80.5, 77.0763)
  point P1665 (83, 72.7461)
  point P1666 (78, 72.7461)
  point P1667 (78, 72.7461)
  point P1668 (90, 72.7461)
  point P1669 (90, 72.7461)
  point P1670 (92.5, 77.0763)
  point P1671 (95, 72.7461)
  point P1672 (90, 72.7461)
  point P1673 (90, 72.7461)
  point P1674 (102, 72.7461)
  point P1675 (102, 72.7461)
  point P1676 (104.5, 77.0763)
  point P1677 (107, 72.7461)
  point P1678 (102, 72.7461)
  point P1679 (102, 72.7461)
  point P1680 (114, 72.7461)
  point P1681 (114, 72.7461)
  point P1682 (116.5, 77.0763)
  point P1683 (119, 72.7461)
  point P1684 (114, 72.7461)
  point P1685 (114, 72.7461)
  point P1686 (126, 72.7461)
  point P1687 (126, 72.7461)
  point P1688 (128.5, 77.0763)
  point P1689 (131, 72.7461)
  point P1690 (126, 72.7461)
  point P1691 (126, 72.7461)
  point P1692 (138, 72.7461)
  point P1693 (138, 72.7461)
  point P1694 (140.5, 77.0763)
  point P1695 (143, 72.7461)
  point P1696 (138, 72.7461)
  point P1697 (138, 72.7461)
  point P1698 (150, 72.7461)
  point P1699 (150, 72.7461)
  point P1700 (152.5, 77.0763)
  point P1701 (155, 72.7461)
  point P1702 (150, 72.7461)
  point P1703 (150, 72.7461)
  dimension "d39" = 5
  dimension "d42" = 12
  dimension "d43" = 12
  constraint coincident L12.start L13.start
  constraint midpoint L11 L12.end
  constraint midpoint L6 L13.end
  measures "d39" distance of L12.start L11
extrude "Extrude5" add sketch "hex" along normal blind 2 contours A0 L0 A1 L1 A2 L2 A3 L3 A4 L4 A5 L5 L74 L75 L76 L80 L81 L82 L83 L86 L87 L88 L89 L92 L93 L94 L95 L98 L99 L100 L101 L104 L105 L107 L182 L183 L184 L187 L218 L219 L221 L222 L290 L291 L292 L295 L332 L333 L335 L336 L398 L399 L400 L401 L403 L446 L447 L448 L449 L450 L501 L502 L506 L507 L508 L509 L510 L511 L560 L561 L562 L563 L564 L565 L566 L569 L614 L615 L616 L618 L619 L674 L675 L677 L678 L679 L723 L724 L727 L788 L791 L792 L836 L837 L838 L840 L841 L890 L891 L893 L894 L895 L939 L940 L943 L1004 L1007 L1008 L1052 L1053 L1054 L1056 L1057 L1112 L1113 L1115 L1116 L1117 L1161 L1162 L1165 L1226 L1229 L1230 L1274 L1275 L1276 L1278 L1279 L1334 L1335 L1337 L1338 L1339 L1383 L1384 L1387 L1448 L1451 L1452 L1496 L1497 L1498 L1500 L1501 L1556 L1557 L1559 L1560 L1561 L1606 L1609 L1612 L1613 L1614 L1615 L1618 L1619 L1620 L1621 L1624 L1625 L1626 L1627 L1630 L1631 L1632 L1633 L1636 L1637 L1638 L1639 L1642 L1643 L1644 L1645 L1648 L1649 L1650 L1651 L1654 L1655 L1656 L1657 L1660 L1661 L1662 L1663 L1666 L1667 L1668 L1669 L1673 L1674 bodies 1
sketch "Sketch8" plane through (0, 0, 0) normal (0, 0, 1) x (1, 0, 0)
  arc A0 (-55, 75) -> (-65, 65) centre (-55, 65) ccw
  line L0 (-55, 75) -> (55, 75)
  arc A1 (65, 65) -> (55, 75) centre (55, 65) ccw
  line L1 (65, 65) -> (65, -20.4398)
  arc A2 (62.1513, -28.5609) -> (65, -20.4398) centre (52, -20.4398) ccw
  line L2 (62.1513, -28.5609) -> (28.9032, -70.121)
  arc A3 (18.7519, -75) -> (28.9032, -70.121) centre (18.7519, -62) ccw
  line L3 (18.7519, -75) -> (-18.7519, -75)
  arc A4 (-28.9032, -70.121) -> (-18.7519, -75) centre (-18.7519, -62) ccw
  line L4 (-28.9032, -70.121) -> (-62.1513, -28.5609)
  arc A5 (-65, -20.4398) -> (-62.1513, -28.5609) centre (-52, -20.4398) ccw
  line L5 (-65, -20.4398) -> (-65, 65)
extrude "Extrude6" add sketch "Sketch8" along normal blind 1 bodies 1
extrude "Extrude7" add sketch "Sketch5" along normal blind 2 separate body contours L9 A30 A31 L31 L32 L33 A34 A35 | L26 L27 L28 L29 A26 A27 A28 A29 L34 A37 L35 L36 L37 A39 makes body 2 at (-71.6445, -15.686, 0) makes body 3 at (71.6445, -15.686, 0)
extrude "Extrude8" add sketch "Sketch5" along normal blind 2 separate body contours L11 A40 L38 A41 L39 A42 L40 A43 L41 L42 | L9 L43 A47 L44 L45 A48 L46 A50 L47 A51 makes body 4 at (71.6445, 62.314, 0) makes body 5 at (-71.6445, 62.314, 0)
sketch "Sketch9" plane through (0, 0, 0) normal (0, 0, 1) x (1, 0, 0)
  line L0 (-30, 50) -> (30, 50)
  line L1 (30, 50) -> (30, -5)
  line L2 (30, -5) -> (-30, -5)
  line L3 (-30, -5) -> (-30, 50)
  dimension "d75" = 60
  dimension "d76" = 55
  constraint horizontal L0
  constraint vertical L1
  constraint horizontal L2
  constraint vertical L3
  measures "d75" distance of L0.start L0.end
  measures "d76" distance of L0.start L2.end
extrude "Extrude9" add sketch "Sketch9" along normal blind 40 separate body makes body 6
extrude "Extrude10" cut 1 faces at (-10, 31.6667, 40) along direction (0, 0, -1) blind 20 on bodies 6 bodies 6
sketch "Sketch10" plane through (0, 0, 0) normal (0, 0, 1) x (1, 0, 0)
hidden bodies 6
